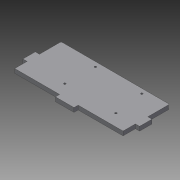
# Autodesk Inventor part: Mount_Mega_Bottom
Saved by Autodesk Inventor 2014 (Build 180170000, 170)
## iProperties
Created: 2014-10-26
Part Number: Mount_Mega_Bottom
Material: Generic
Document SubType Name: Modeling
Designer: ThatOtherGuy
Density: 1 g/cm^3
Appearance: Default
Author: ThatOtherGuy
Autodesk Inventor part; units mm, degrees
ref_plane "YZ Plane" through (0, 0, 0) normal (1, 0, 0) x (0, 1, 0)
ref_plane "XZ Plane" through (0, 0, 0) normal (0, 1, 0) x (-1, 0, 0)
ref_plane "XY Plane" through (0, 0, 0) normal (0, 0, 1) x (1, 0, 0)
sketch "Sketch1" plane through (0, 0, 0) normal (0, 0, 1) x (1, 0, 0)
  line L0 (0, 0) -> (175, 0)
  line L1 (175, 0) -> (175, 75)
  line L2 (175, 75) -> (0, 75)
  line L3 (0, 75) -> (0, 0)
  dimension "d0" = 175
  dimension "d1" = 75
  constraints: 8 end point, 2 parallel, 1 horizontal, 1 perpendicular
  measures "d0" distance of L0.start L0.end
  measures "d1" distance of L2.end L0.start
extrude "Extrusion1" add sketch "Sketch1" along normal blind 6.731
sketch "Sketch2" plane through (0, 0, 6.731) normal (0, 0, 1) x (1, 0, 0)
  line L0 (0, 0) -> (175, 0) projected
  line L1 (175, 0) -> (175, 75) projected
  line L2 (175, 75) -> (0, 75) projected
  line L3 (0, 75) -> (0, 0) projected
  line L4 (61.6333, 19.24) -> (144.1833, 19.24)
  line L5 (144.1833, 19.24) -> (144.1833, 67.5)
  line L6 (144.1833, 67.5) -> (137.8333, 67.5)
  line L7 (137.8333, 67.5) -> (62.9033, 67.5)
  line L8 (62.9033, 67.5) -> (61.6333, 67.5)
  line L9 (61.6333, 67.5) -> (61.6333, 19.24)
  dimension "d9" = 1.27
  dimension "d10" = 48.26
  dimension "d12" = 82.55
  dimension "d13" = 74.93
  dimension "d15" = 61.6333
  dimension "d16" = 30.8167
  dimension "d17" = 7.5
  constraints: 12 end point, 2 coincident, 2 collinear, 2 parallel, 2 perpendicular
  measures "d9" distance of L7.end L8.end
  measures "d10" distance of L8.end L4.start
  measures "d12" distance of L4.start L4.end
  measures "d13" distance of L6.end L7.end
  measures "d15" distance between parallel lines of L3 L9
  measures "d16" distance between parallel lines of L1 L5
  measures "d17" distance between parallel lines of L2 L7
hole "Hole1" at (62.9033, 67.5, 6.731) at (144.1833, 19.24, 6.731) at (61.6333, 19.24, 6.731) at (137.8333, 67.5, 6.731) direction (0, 0, -1) diameter 3.176 end through all
sketch "Sketch3" plane through (0, 0, 6.731) normal (0, 0, 1) x (1, 0, 0)
  line L0 (0, 0) -> (175, 0) projected
  line L1 (175, 0) -> (175, 75) projected
  line L2 (0, 75) -> (0, 0) projected
  line L3 (72.5, 0) -> (102.5, 0)
  line L4 (102.5, 0) -> (102.5, -6.731)
  line L5 (102.5, -6.731) -> (72.5, -6.731)
  line L6 (72.5, -6.731) -> (72.5, 0)
  line L7 (0, 40) -> (-6.731, 40)
  line L8 (-6.731, 40) -> (-6.731, 20)
  line L9 (-6.731, 20) -> (0, 20)
  line L10 (0, 20) -> (0, 40)
  line L11 (175, 40) -> (181.731, 40)
  line L12 (181.731, 40) -> (181.731, 20)
  line L13 (181.731, 20) -> (175, 20)
  line L14 (175, 20) -> (175, 40)
  point P0 (87.5, -6.731)
  point P1 (87.5, 0)
  point P2 (-6.731, 30)
  point P3 (181.731, 30)
  dimension "d25" = 6.731
  dimension "d26" = 30
  dimension "d29" = 20
  dimension "d31" = 20
  constraints: 24 end point, 6 parallel, 4 midpoint, 3 equal length, 3 horizontal, 3 perpendicular, 3 point on line, 1 horizontal alignment, 1 vertical alignment
  measures "d25" distance of L5.end L3.start
  measures "d26" distance of L4.end L5.end
  measures "d29" distance of L7.end L8.end
  measures "d31" distance between parallel lines of L0 L9
extrude "Extrusion2" add sketch "Sketch3" against normal blind 6.731
fillet "Fillet1" radius 2 2 edges at (0, 75, 3.3655) (175, 75, 3.3655)
equation "\"d7\" = THICKB"
equation "\"d15\" = 2 * d16"
equation "\"d25\" = THICKB"
equation "\"d27\" = THICKB"
equation "\"THICKA\" = 3.175"
equation "\"THICKB\" = 6.731"
equation "\"THICKC\" = 12.7"
equation "\"THICKPLY\" = 5"
equation "\"MAGDIA\" = 9.5"
equation "\"BALLDIA\" = 12"
body "Solid1"
